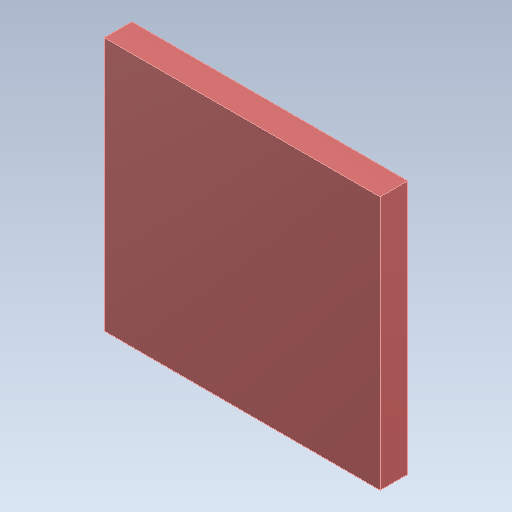
# Autodesk Inventor part: W237-102
Saved by Autodesk Inventor 2021 (Build 250183000, 183)
## iProperties
Created: 2020-11-18
Part Number: W237-102
Material: Generic
Document SubType Name: Modeling
Designer: Admin
Density: 1 g/cm^3
Appearance: W237-102, W237-102
Author: Admin
Autodesk Inventor part; units mm, degrees
ref_plane "YZ Plane" through (0, 0, 0) normal (1, 0, 0) x (0, 1, 0)
ref_plane "XZ Plane" through (0, 0, 0) normal (0, 1, 0) x (-1, 0, 0)
ref_plane "XY Plane" through (0, 0, 0) normal (0, 0, 1) x (1, 0, 0)
sketch "W237-102, W237-102_63" plane through (0, 0, 0) normal (0, 0, 1) x (1, 0, 0)
  line L0 (-4.989, 3.734) -> (4.993, 3.734)
  line L1 (4.993, 3.734) -> (4.993, -5.461)
  line L2 (4.993, -5.461) -> (-4.989, -5.461)
  line L3 (-4.989, -5.461) -> (-4.989, 3.734)
  constraints: 8 end point
extrude "Extrusion1" add sketch "W237-102, W237-102_63" along normal blind 1
body "Solid1"
